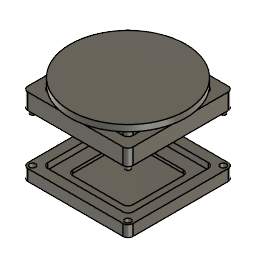
capteur boîte (Autodesk Fusion 360 design; units mm, degrees)
Autodesk Fusion 360 part; units mm, degrees
sketch "Sketch1" plane through (0, 0, 0) normal (0, 0, 1) x (1, 0, 0) in component "Base"
  line L0 (17, -17) -> (-17, -17)
  line L1 (-17, -17) -> (-17, 17)
  line L2 (-17, 17) -> (17, 17)
  line L3 (17, 17) -> (17, -17)
  line L4 (17, -17) -> (-17, 17) construction
  line L5 (-17, -17) -> (17, 17) construction
  line L6 (-21, -21) -> (-21, 21)
  line L7 (-21, 21) -> (21, 21)
  line L8 (21, 21) -> (21, -21)
  line L9 (21, -21) -> (-21, -21)
  line L10 (12, -12) -> (-12, -12)
  line L11 (-12, -12) -> (-12, 12)
  line L12 (-12, 12) -> (12, 12)
  line L13 (12, 12) -> (12, -12)
  line L14 (12, -12) -> (-12, 12) construction
  line L15 (-12, -12) -> (12, 12) construction
  line L16 (2.5, 21) -> (2.5, 17)
  line L17 (-2.5, 21) -> (-2.5, 17)
  circle A0 centre (-19, 19) radius 1.2
  circle A1 centre (-19, 19) radius 1.2
  circle A2 centre (-19, 19) radius 1
  circle A3 centre (19, 19) radius 1.2
  circle A4 centre (19, 19) radius 1
  circle A5 centre (19, 19) radius 1.2
  circle A6 centre (-19, -19) radius 1.2
  circle A7 centre (-19, -19) radius 1.2
  circle A8 centre (-19, -19) radius 1
  circle A9 centre (19, -19) radius 1.2
  circle A10 centre (19, -19) radius 1.2
  circle A11 centre (19, -19) radius 1
  line L18 (15.8, -15.8) -> (-15.8, -15.8)
  line L19 (-15.8, -15.8) -> (-15.8, 15.8)
  line L20 (-15.8, 15.8) -> (15.8, 15.8)
  line L21 (15.8, 15.8) -> (15.8, -15.8)
  line L22 (-10, 15.8) -> (-10, 17)
  line L23 (10, 15.8) -> (10, 17)
  line L24 (0, -17) -> (0, -15.8) construction
  line L25 (-10, -17) -> (-10, -15.8)
  line L26 (10, -17) -> (10, -15.8)
  dimension "d1" = 34
  dimension "d2" = 34
  dimension "d3" = -4
  dimension "d4" = 24
  dimension "d5" = 24
  dimension "d6" = 5
  dimension "d7" = 2.4
  dimension "d8" = 2.4
  dimension "d9" = -0.2
  dimension "d10" = -0.2
  dimension "d11" = 2.4
  dimension "d12" = 2.4
  dimension "d13" = -0.2
  dimension "d14" = 2.4
  dimension "d15" = 2.4
  dimension "d16" = -0.2
  dimension "d17" = 2.4
  dimension "d18" = 2.4
  dimension "d19" = 1.2
  dimension "d20" = 20
  dimension "d37" = 20
  constraint perpendicular L0 L1
  constraint parallel L0 L2
  constraint parallel L1 L3
  constraint horizontal L0
  constraint coincident L4 origin
  constraint coincident L5 origin
  constraint perpendicular L10 L11
  constraint parallel L10 L12
  constraint parallel L11 L13
  constraint horizontal L10
  constraint coincident L14 origin
  constraint coincident L15 origin
  constraint coincident L7 L16.start
  constraint coincident L2 L16.end
  constraint perpendicular L7 L16
  constraint coincident L7 L17.start
  constraint coincident L2 L17.end
  constraint perpendicular L2 L17
  constraint coincident L20 L22.start
  constraint coincident L2 L22.end
  constraint perpendicular L2 L22
  constraint coincident L20 L23.start
  constraint coincident L2 L23.end
  constraint perpendicular L2 L23
  constraint midpoint L0 L24.start
  constraint midpoint L18 L24.end
  constraint perpendicular L18 L24
  constraint coincident L0 L25.start
  constraint coincident L18 L25.end
  constraint perpendicular L18 L25
  constraint coincident L0 L26.start
  constraint coincident L18 L26.end
  constraint perpendicular L18 L26
  constraint symmetric L24 L25 L26
  measures "d1" distance of L1.end L2.end
  measures "d2" distance of L0.end L1.end
  measures "d4" distance of L11.end L12.end
  measures "d5" distance of L10.end L11.end
  measures "d6" distance of L16 L17
  measures "d7" diameter of A0
  measures "d8" diameter of A1
  measures "d11" diameter of A3
  measures "d12" diameter of A5
  measures "d14" diameter of A7
  measures "d15" diameter of A6
  measures "d17" diameter of A10
  measures "d18" diameter of A9
  measures "d20" distance of L22 L23
  measures "d37" distance of L25 L26
extrude "Extrude1" add sketch "Sketch1" against normal blind 0.8 contours L0 L1 L2 L3 L6 L7 L8 L9 L16 L17 | L0 L2 L3 L18 L20 L21 L23 L26 | L0 L18 L25 L26 | L0 L1 L2 L18 L19 L20 L22 L25 | L18 L19 L20 L21 | L2 L20 L22 L23 | L2 L7 L16 L17 | L10 L11 L12 L13 | A0 A1 | A2 | A3 A5 | A4 | A6 A7 | A8 | A9 A10 | A11 makes body 1 in component "Base"
extrude "Extrude2" add sketch "Sketch1" along normal blind 1.2 contours L0 L1 L2 L3 L6 L7 L8 L9 L16 L17 | L0 L2 L3 L18 L20 L21 L23 L26 | L0 L18 L25 L26 | L0 L1 L2 L18 L19 L20 L22 L25 | L18 L19 L20 L21 | L2 L20 L22 L23 | L2 L7 L16 L17 | A0 A1 | A2 | A3 A5 | A4 | A6 A7 | A8 | A9 A10 | A11 bodies 1 in component "Base"
extrude "Extrude3" add sketch "Sketch1" along normal blind 2.5 from surface at 1.2 contours L0 L1 L2 L3 L6 L7 L8 L9 L16 L17 | L2 L7 L16 L17 | A0 A1 | A2 | A3 A5 | A4 | A6 A7 | A8 | A9 A10 | A11 bodies 1 in component "Base"
extrude "Extrude4" cut sketch "Sketch1" against normal blind 2.2 from surface at 3.7 contours A0 A1 | A2 | A3 A5 | A4 | A6 A7 | A8 | A9 A10 | A11 bodies 1 in component "Base"
extrude "Extrude1'" add sketch "Sketch1" along normal blind 6.4 from surface at -0.8 separate body contours L0 L1 L2 L3 L6 L7 L8 L9 L16 L17 | L2 L7 L16 L17 | A0 A1 | A2 | A3 A5 | A4 | A6 A7 | A8 | A9 A10 | A11 makes body 2 in component "Tampa"
extrude "Extrude2'" add sketch "Sketch1" against normal blind 1.2 from surface at 5.6 separate body contours L0 L18 L25 L26 | L18 L19 L20 L21 | L10 L11 L12 L13 makes body 3 in component "Tampa"
extrude "Extrude3'" cut sketch "Sketch1" along normal blind 1.4 from surface at -0.8 contours L2 L7 L16 L17 bodies 2 in component "Tampa"
extrude "Extrude4'" add sketch "Sketch1" against normal blind 2 from surface at -0.8 contours A2 | A4 | A8 | A11 bodies 2 in component "Tampa"
combine "Combine1" operation add target body 2 tool bodies 3 in component "Tampa"
fillet "Fillet1" radius 2 12 edges at (21, 21, 2.4) (21, -21, 2.4) (-21, -21, 2.4) (-21, 21, 2.4) (-15.8, 15.8, 5) (15.8, 15.8, 5) (15.8, -15.8, 5) (-15.8, -15.8, 5) (-17, -17, 2.4) (-17, 17, 2.4) (17, 17, 2.4) (17, -17, 2.4) on bodies 2 in component "Tampa"
fillet "Fillet1" radius 2 2 edges at (2.5, 17, -0.1) (-2.5, 17, -0.1) on bodies 2 in component "Tampa"
fillet "Fillet1'" radius 2 11 edges at (17, -17, 2.45) (-17, -17, 2.45) (-12, 12, 0.6) (-12, -12, 0.6) (12, -12, 0.6) (17, 17, 2.45) (12, 12, 0.6) (-21, -21, 1.45) (21, -21, 1.45) (21, 21, 1.45) (-21, 21, 1.45) on bodies 1 in component "Base"
fillet "Fillet1'" radius 2 1 edges at (-17, 17, 2.45) on bodies 1 in component "Base"
move_body "Déplacer1" bodies 2 to x (1, 0, 0) y (0, 1, 0) z (0, 0, 1) at (0, 0, 20) in component "Tampa"
sketch "Esquisse2" plane through (0, 0, 30.1) normal (0, 0, 1) x (-1, 0, 0)
  arc A0 (19, -21) -> (21, -19) centre (19, -19) ccw
  line L0 (21, -19) -> (21, 19)
  arc A1 (21, 19) -> (19, 21) centre (19, 19) ccw
  line L1 (19, 21) -> (-19, 21)
  arc A2 (-19, 21) -> (-21, 19) centre (-19, 19) ccw
  line L2 (-21, 19) -> (-21, -19)
  arc A3 (-21, -19) -> (-19, -21) centre (-19, -19) ccw
  line L3 (-19, -21) -> (19, -21)
  arc A4 (15.8, 13.8) -> (13.8, 15.8) centre (13.8, 13.8) ccw
  line L4 (13.8, 15.8) -> (10, 15.8)
  line L5 (10, 15.8) -> (10, 17)
  line L6 (10, 17) -> (15, 17)
  arc A5 (17, 15) -> (15, 17) centre (15, 15) ccw
  line L7 (17, 15) -> (17, -15)
  arc A6 (15, -17) -> (17, -15) centre (15, -15) ccw
  line L8 (15, -17) -> (-15, -17)
  arc A7 (-17, -15) -> (-15, -17) centre (-15, -15) ccw
  line L9 (-17, -15) -> (-17, 15)
  arc A8 (-15, 17) -> (-17, 15) centre (-15, 15) ccw
  line L10 (-15, 17) -> (-10, 17)
  line L11 (-10, 17) -> (-10, 15.8)
  line L12 (-10, 15.8) -> (-13.8, 15.8)
  arc A9 (-13.8, 15.8) -> (-15.8, 13.8) centre (-13.8, 13.8) ccw
  line L13 (-15.8, 13.8) -> (-15.8, -13.8)
  arc A10 (-15.8, -13.8) -> (-13.8, -15.8) centre (-13.8, -13.8) ccw
  line L14 (-13.8, -15.8) -> (13.8, -15.8)
  arc A11 (13.8, -15.8) -> (15.8, -13.8) centre (13.8, -13.8) ccw
  line L15 (15.8, -13.8) -> (15.8, 13.8)
  line L16 (10, 15.8) -> (-10, 15.8)
  constraint coincident L4.end L5.start
  constraint coincident L11.end L12.start
extrude "Extrusion5" add sketch "Esquisse2" along normal blind 4 contours A4 L4 L12 A9 L13 A10 L14 A11 L15 L16 sketch seen with x (1, 0, 0) y (0, 1, 0) z (0, 0, 1) at (0, 0, -4.5) bodies 2 in component "Tampa"
sketch "Esquisse3" plane through (0, 0, 34.1) normal (0, 0, 1) x (-1, 0, 0)
  line L0 (13.8, 15.8) -> (-13.8, 15.8)
  arc A0 (-13.8, 15.8) -> (-15.8, 13.8) centre (-13.8, 13.8) ccw
  line L1 (-15.8, 13.8) -> (-15.8, -13.8)
  arc A1 (-15.8, -13.8) -> (-13.8, -15.8) centre (-13.8, -13.8) ccw
  line L2 (-13.8, -15.8) -> (13.8, -15.8)
  arc A2 (13.8, -15.8) -> (15.8, -13.8) centre (13.8, -13.8) ccw
  line L3 (15.8, -13.8) -> (15.8, 13.8)
  arc A3 (15.8, 13.8) -> (13.8, 15.8) centre (13.8, 13.8) ccw
  circle A4 centre (0, 0) radius 23
  dimension "d66" = 46
  constraint coincident A4.centre origin
  measures "d66" diameter of A4
extrude "Extrusion6" add sketch "Esquisse3" against normal blind 2.5 contours L0 A0 L1 A1 L2 A2 L3 A3 | A4 sketch seen with x (1, 0, 0) y (0, 1, 0) z (0, 0, 1) at (0, 0, -4.5) bodies 2 in component "Tampa"
component "Base" placed x (1, 0, 0) y (0, 1, 0) z (0, 0, 1) at (0, 0, 0)
component "Tampa" placed x (1, 0, 0) y (0, 1, 0) z (0, 0, 1) at (0, 0, 4.5)
